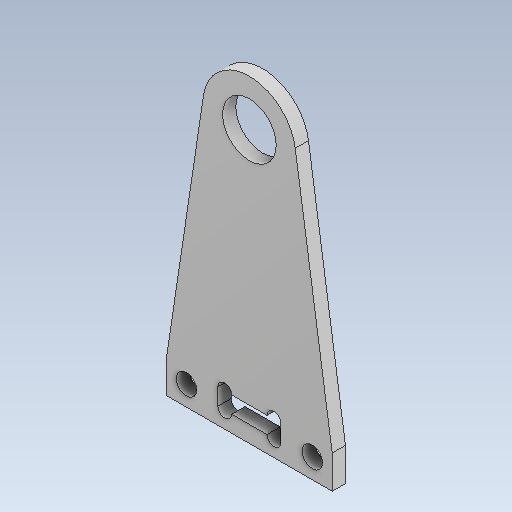
# Autodesk Inventor part: Foot_front_frame
Saved by Autodesk Inventor 2020 (Build 240168000, 168)
## iProperties
Created: 2021-09-15
Part Number: Foot_front_frame
Material: アルミニウム 2014-T4
Document SubType Name: Modeling
Designer: Naoki Iwasawa
Density: 2.8 g/cm^3
Appearance: 滑らか - 淡い灰色
Description: A2017 T2
Mass: 4.5322 g
Surface Area: 20.2588 cm^2
Volume: 1.61864 cm^3
Author: Naoki Iwasawa
Autodesk Inventor part; units mm, degrees
ref_plane "YZ Plane" through (0, 0, 0) normal (1, 0, 0) x (0, 1, 0)
ref_plane "XZ Plane" through (0, 0, 0) normal (0, 1, 0) x (-1, 0, 0)
ref_plane "XY Plane" through (0, 0, 0) normal (0, 0, 1) x (1, 0, 0)
derived "Foot_back_frame.ipt"
sketch "スケッチ1" plane through (0, 0, 0) normal (0, 0, 1) x (1, 0, 0)
  line L0 (-63.6765, 0) -> (66.53, 0) construction
  line L1 (0, 73.5962) -> (0, -63.7716) construction
  circle A0 centre (0, 0) radius 5.05 construction
  circle A1 centre (0, 0) radius 8 construction
  circle A2 centre (0, 0) radius 10.9 construction
  circle A3 centre (0, 8.5) radius 1.35 construction
  circle A4 centre (0, 8.5) radius 2.4 construction
  circle A5 centre (-8.5, 0) radius 2.4 construction
  circle A6 centre (-8.5, 0) radius 1.35 construction
  circle A7 centre (0, -8.5) radius 2.4 construction
  circle A8 centre (0, -8.5) radius 1.35 construction
  circle A9 centre (8.5, 0) radius 2.4 construction
  circle A10 centre (8.5, 0) radius 1.35 construction
  line L2 (12.5, -41) -> (-12.5, -41)
  line L3 (-12.5, -41) -> (-12.5, -36)
  line L4 (-12.5, -36) -> (12.5, -36)
  line L5 (12.5, -36) -> (12.5, -41)
  line L6 (12.5, -41) -> (-12.5, -36) construction
  line L7 (-12.5, -41) -> (12.5, -36) construction
  line L8 (12.5, -36) -> (10.8894, 0.4808) construction
  line L9 (-12.5, -36) -> (-10.8894, 0.4808) construction
  circle A11 centre (-9.5, -38) radius 1.55
  line L10 (-12.5, -38) -> (12.5, -38) construction
  line L11 (-4.75, -36) -> (-4.75, -41)
  line L12 (4.75, -36) -> (4.75, -41) construction
  circle A12 centre (9.5, -38) radius 1.55
  line L13 (-4.75, -36) -> (4.75, -36)
  line L14 (4.75, -36) -> (4.75, -38.5)
  line L15 (4.75, -38.5) -> (-4.75, -38.5)
  line L16 (-4.75, -38.5) -> (-4.75, -36) construction
  circle A13 centre (0, 0) radius 7
  circle A14 centre (0, 0) radius 4.05
  line L17 (-12.5, -36) -> (12.5, -36)
  line L18 (12.5, -36) -> (12.5, -41)
  line L19 (12.5, -41) -> (-12.5, -41)
  line L20 (-12.5, -41) -> (-12.5, -36)
  line L21 (-12.5, -36) -> (-9.007, -12.804)
  line L22 (12.5, -36) -> (6.922, 1.0423)
  line L23 (-4.75, -36) -> (4.75, -36)
  line L24 (-4.75, -37.25) -> (4.75, -37.25) construction
  line L25 (-9.007, -12.804) -> (-6.922, 1.0423)
  line L26 (-4.76, -38.51) -> (4.76, -38.51)
  line L27 (4.76, -38.51) -> (4.76, -35.99)
  line L28 (4.76, -35.99) -> (-4.76, -35.99)
  line L29 (-4.76, -35.99) -> (-4.76, -38.51)
  circle A15 centre (-3.71, -35.99) radius 1.05
  circle A16 centre (-3.71, -38.51) radius 1.05
  circle A17 centre (3.71, -38.51) radius 1.05
  circle A18 centre (3.71, -35.99) radius 1.05
  point P0 (0, -38.5)
  point P1 (4.75, -36)
  point P2 (7.9399, 0.9791)
  point P3 (-7.9399, 0.9791)
  point P4 (-6.922, 1.0423)
  point P5 (2.66, -38.51)
  point P6 (-2.66, -38.51)
  point P7 (-2.66, -35.99)
  point P8 (2.66, -35.99)
  point P9 (-4.75, -38.5)
  dimension "d3" = 14
  dimension "d4" = 8.1
  measures "d3" diameter of A13
  measures "d4" diameter of A14
extrude "押し出し1" add sketch "スケッチ1" along normal blind 2 contours L2 L11 A16 L26 A17 L27 L4 L5 | L2 L3 L4 L29 A16 L11 | L4 L27 A18 L28 A15 L29 L21 L25 A13 L22 | A13
